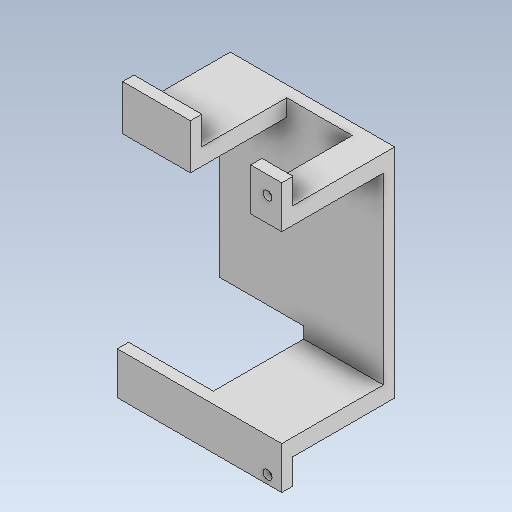
# Autodesk Inventor part: tray
Saved by Autodesk Inventor 2020 (Build 240168000, 168)
## iProperties
Created: 2022-07-07
Part Number: tray
Material: 일반
Document SubType Name: Modeling
Designer: SeungJin
Density: 1 g/cm^3
Appearance: 기본값
Author: SeungJin
Autodesk Inventor part; units mm, degrees
ref_plane "YZ Plane" through (0, 0, 0) normal (1, 0, 0) x (0, 1, 0)
ref_plane "XZ Plane" through (0, 0, 0) normal (0, 1, 0) x (-1, 0, 0)
ref_plane "XY Plane" through (0, 0, 0) normal (0, 0, 1) x (1, 0, 0)
sketch "스케치1" plane through (0, 0, 0) normal (0, 0, 1) x (1, 0, 0)
  circle A0 centre (-12.5, -15) radius 2.067 projected
  line L0 (-145.5, 0) -> (0, 0) projected
  line L1 (-145.5, 0) -> (-145.5, -25) projected
  line L2 (0, -25) -> (-145.5, -25) projected
  line L3 (0, 0) -> (0, -25) projected
  circle A1 centre (-12.5, -35) radius 2.067 projected
  line L4 (0, -50) -> (-145.5, -50) projected
  line L5 (0, -50) -> (0, -25) projected
  line L6 (-145.5, -25) -> (0, -25) projected
  line L7 (-145.5, -50) -> (-145.5, -25) projected
  line L8 (-27.5, 192.5) -> (-60.5, 192.5) projected
  line L9 (-27.5, 192.5) -> (-27.5, 217.5) projected
  line L10 (-60.5, 217.5) -> (-27.5, 217.5) projected
  line L11 (-60.5, 192.5) -> (-60.5, 217.5) projected
  circle A2 centre (25, 206.5) radius 4.188 projected
  circle A3 centre (-12.5, 199) radius 2.067 projected
  circle A4 centre (-12.5, 211) radius 2.067 projected
  line L12 (42.5, 192.5) -> (-27.5, 192.5) projected
  line L13 (42.5, 192.5) -> (42.5, 217.5) projected
  line L14 (-27.5, 217.5) -> (42.5, 217.5) projected
  line L15 (-27.5, 192.5) -> (-27.5, 217.5) projected
  line L16 (0, 0) -> (-145.5, 0)
  line L17 (-145.5, 0) -> (-145.5, 15)
  line L18 (-145.5, 15) -> (0, 15)
  line L19 (0, 15) -> (0, 0)
  line L20 (42.5, 192.5) -> (-27.5, 192.5)
  line L21 (-27.5, 192.5) -> (-27.5, 177.5)
  line L22 (-27.5, 177.5) -> (42.5, 177.5)
  line L23 (42.5, 177.5) -> (42.5, 192.5)
  line L24 (0, 192.5) -> (0, 217.5) projected
  line L25 (0, 177.5) -> (0, 217.5)
  line L26 (0, -50) -> (-145.5, -50)
  line L27 (-145.5, -50) -> (-145.5, -65)
  line L28 (-145.5, -65) -> (0, -65)
  line L29 (0, -65) -> (0, -50)
  line L30 (-27.5, 215) -> (42.5, 215)
  line L31 (-145.5, -22.5) -> (0, -22.5)
  point P0 (0, 215)
  dimension "d0" = 15
  dimension "d1" = 15
  dimension "d37" = 15
  dimension "d64" = 2.5
  constraints: 30 end point, 6 parallel, 6 perpendicular, 5 point on line, 3 horizontal
  measures "d0" distance of L16.end L17.end
  measures "d1" distance of L21.end L20.end
  measures "d37" distance of L27.end L26.end
  measures "d64" distance between parallel lines of L31 L2
extrude "돌출1" add sketch "스케치1" along normal blind 10 contours A0 | L17 L18 L19 L0 | L0 L3 L31 L1 | L9 L30 L24 L12 | L12 L25 L22 L21 | A3 | A4
ref_plane "작업 평면2" through (-45, 217.5, -4.7) normal (0, 0, 1) x (0, 1, 0)
sketch "스케치8" plane through (-45, 217.5, -4.7) normal (0, 0, 1) x (0, 1, 0)
  line L0 (0, 0) -> (0, 281)
  line L1 (0, 281) -> (-25, 281)
  line L2 (-25, 0) -> (-25, 281)
  line L3 (0, 0) -> (-25, 0)
  line L4 (-25, 20) -> (0, 20)
  line L5 (0, 140.5) -> (0, 90.5)
  line L6 (0, 90.5) -> (-25, 90.5)
  line L7 (-25, 90.5) -> (-25, 140.5)
  line L8 (-25, 90.5) -> (-25, 140.5)
  line L9 (-25, 90.5) -> (0, 90.5)
  line L10 (0, 90.5) -> (0, 40.5)
  line L11 (0, 40.5) -> (-25, 40.5)
  line L12 (-25, 40.5) -> (-25, 90.5)
  line L13 (-25, 90.5) -> (-40, 90.5)
  line L14 (-40, 90.5) -> (-40, 40.5)
  line L15 (-40, 40.5) -> (-25, 40.5)
  line L16 (-25, 40.5) -> (-25, 90.5)
  line L17 (163.5, 100.5) -> (-286.5, 100.5) projected
  line L18 (0, 100.5) -> (-40, 100.5)
  line L19 (-40, 100.5) -> (-40, 90.5)
  line L20 (-25, 20) -> (-40, 20)
  line L21 (-40, 20) -> (-40, 40.5)
  point P0 (-217.5, -45)
  point P1 (-25, 90.5)
  point P2 (-25, 40.5)
  point P3 (-25, 90.5)
  point P4 (0, 100.5)
  dimension "d28" = 50
  dimension "d29" = 15
  constraints: 42 end point, 6 point on line, 4 perpendicular, 2 parallel, 1 horizontal, 1 midpoint
  measures "d28" distance of L9.end L10.end
  measures "d29" distance of L15.end L14.end
extrude "돌출8" add sketch "스케치8" along normal blind 10 contours L11 L2 L6 L0 | L6 L2 L17 L0 | L15 L14 L13 L2 | L13 L19 L17 L2
ref_plane "작업 평면7" through (0, -50, -80) normal (0, 0, -1) x (-1, 0, 0)
sketch "스케치15" plane through (0, -50, -80) normal (0, 0, -1) x (-1, 0, 0)
  line L0 (70.5, -15) -> (70.5, 50)
  line L1 (70.5, 50) -> (0, 50)
  line L2 (0, 50) -> (0, -15)
  line L3 (0, -15) -> (70.5, -15)
  line L4 (27.5, 227.5) -> (0, 227.5)
  line L5 (27.5, 242.5) -> (27.5, 227.5)
  line L6 (0, 242.5) -> (27.5, 242.5)
  line L7 (0, 227.5) -> (0, 242.5)
  line L8 (145.5, 227.5) -> (85.5, 227.5)
  line L9 (145.5, 242.5) -> (145.5, 227.5)
  line L10 (85.5, 242.5) -> (145.5, 242.5)
  line L11 (85.5, 227.5) -> (85.5, 242.5)
  line L12 (0, -15) -> (145.5, -15)
  line L13 (145.5, -15) -> (145.5, 242.5)
  line L14 (145.5, 242.5) -> (0, 242.5)
  line L15 (0, 242.5) -> (0, -15)
  line L16 (0, 50) -> (145.5, 50)
  circle A0 centre (93.5, 13) radius 2.067
  circle A1 centre (93.5, 37) radius 2.067
  circle A2 centre (147.5, 37) radius 2.067
  circle A3 centre (147.5, 13) radius 2.067
  line L17 (70.5, 0) -> (70.5, 50)
  line L18 (145.5, 50) -> (145.5, 81)
  line L19 (145.5, 75) -> (70.5, 75)
  line L20 (70.5, 50) -> (70.5, 75)
  point P0 (0, 227.5)
  point P1 (85.5, 242.5)
  point P2 (70.5, 25)
  dimension "d54" = 50
  constraints: 42 end point, 4 centre point, 1 midpoint, 1 point on line
  measures "d54" distance from line of L19 point (70.5, 25)
extrude "돌출16" add sketch "스케치15" along normal blind 10 contours L1 L15 L4 L5 L14 L11 L8 L13 L19 L20 | L7 L6 L5 L4 | L8 L11 L10 L9
sketch "스케치16" plane through (0, -50, -80) normal (0, 0, 1) x (1, 0, 0)
  line L0 (-145.5, 75) -> (-145.5, 242.5) projected
  line L1 (-70.5, 75) -> (-145.5, 75) projected
  line L2 (-70.5, 50) -> (-70.5, 75) projected
  line L3 (0, 50) -> (-70.5, 50) projected
  line L4 (0, 242.5) -> (0, 50) projected
  line L5 (-145.5, 242.5) -> (0, 242.5) projected
  line L6 (0, 50) -> (-70.5, 50) projected
  line L7 (-70.5, 50) -> (-70.5, 75) projected
  line L8 (-145.5, 227.5) -> (-85.5, 227.5) projected
  line L9 (-85.5, 227.5) -> (-85.5, 267.5) projected
  line L10 (-27.5, 227.5) -> (0, 227.5) projected
  line L11 (-27.5, 265) -> (-27.5, 227.5) projected
  line L12 (0, 65) -> (-145.5, 65) projected
  point P0 (-27.5, 267.5)
  point P1 (-27.5, 242.5)
  point P2 (-85.5, 242.5)
  point P3 (-70.5, 65)
extrude "돌출17" add sketch "스케치16" along normal up to surface (80 mm away) contours L0 L5 L9 L8 | L12 L4 L3 L2 | L5 L4 L10 L11
sketch "스케치17" plane through (0, 0, 10) normal (0, 0, 1) x (1, 0, 0)
  circle A0 centre (-12.5, 199) radius 2.067 projected
  circle A1 centre (-12.5, 211) radius 2.067 projected
  circle A2 centre (-12.5, -15) radius 2.067 projected
  point P0 (0, 0)
hole "구멍1" at (-12.5, 199, 10) at (-12.5, -15, 10) direction (0, 0, -1) diameter 4.5 end through all counterbore diameter 8 counterbore depth 5 clearance for "Hex Head Cap Screw ISO 24017" size "M4" standard "ISO"
